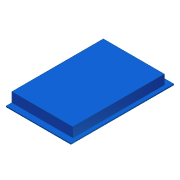
# Autodesk Inventor part: ElectronicsVolume
Saved by Autodesk Inventor 2012 (Build 160160000, 160)
## iProperties
Created: 2013-01-20
Part Number: ElectronicsVolume
Material: Default
Document SubType Name: Modeling
Designer: JesseK
Density: 0.442879 g/cm^3
Mass: 6803.89 g
Surface Area: 7474.18 cm^2
Volume: 15362.9 cm^3
Author: JesseK
Autodesk Inventor part; units mm, degrees
ref_plane "YZ Plane" through (0, 0, 0) normal (1, 0, 0) x (0, 1, 0)
ref_plane "XZ Plane" through (0, 0, 0) normal (0, 1, 0) x (-1, 0, 0)
ref_plane "XY Plane" through (0, 0, 0) normal (0, 0, 1) x (1, 0, 0)
sketch "Sketch1" plane through (0, 0, 0) normal (0, 0, 1) x (1, 0, 0)
  line L0 (0, 0) -> (431.8, 0)
  line L1 (406.4, 69.85) -> (0, 69.85)
  line L2 (0, 69.85) -> (0, 0)
  line L3 (406.4, 69.85) -> (406.4, 6.35)
  line L4 (406.4, 6.35) -> (431.8, 6.35)
  line L5 (431.8, 6.35) -> (431.8, 0)
  dimension "d0" = 69.85
  dimension "d1" = 431.8
  dimension "d2" = 6.35
  dimension "d3" = 25.4
  constraints: 12 end point, 3 vertical, 2 horizontal, 1 parallel
  measures "d0" distance of L1.end L0.start
  measures "d1" distance of L0.start L0.end
  measures "d2" distance of L4.end L0.end
  measures "d3" distance of L3.end L4.end
extrude "Extrusion1" add sketch "Sketch1" along normal blind 685.8
sketch "Sketch2" plane through (0, 0, 0) normal (-1, 0, 0) x (0, 0, 1)
  line L0 (0, 0) -> (685.8, 0) projected
  line L1 (685.8, 69.85) -> (647.7, 69.85)
  line L2 (647.7, 69.85) -> (647.7, 6.35)
  line L3 (647.7, 6.35) -> (685.8, 6.35)
  line L4 (685.8, 6.35) -> (685.8, 69.85)
  line L5 (0, 69.85) -> (38.1, 69.85)
  line L6 (38.1, 69.85) -> (38.1, 6.35)
  line L7 (38.1, 6.35) -> (0, 6.35)
  line L8 (0, 6.35) -> (0, 69.85)
  dimension "d6" = 6.35
  dimension "d7" = 38.1
  constraints: 16 end point, 4 parallel, 2 equal length, 2 horizontal, 2 perpendicular
  measures "d6" distance between parallel lines of L0 L3
  measures "d7" distance of L2.end L3.end
extrude "Extrusion2" cut sketch "Sketch2" against normal through all
body "Solid1"
